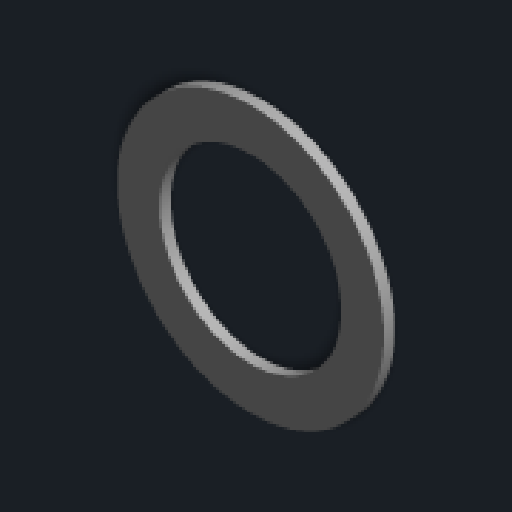
# Autodesk Inventor part: NeckRingAlign
Saved by Autodesk Inventor 2025.2 (Build 292293000, 293)
## iProperties
Created: 2025-09-16
Part Number: NeckRingAlign
Material: Generic
Document SubType Name: Sheet Metal
Designer: valer
Density: 1 g/cm^3
Sheet Metal Rule: Default_mm
Appearance: Default
Author: valer
Autodesk Inventor part; units mm, degrees
ref_plane "YZ Plane" through (0, 0, 0) normal (1, 0, 0) x (0, 1, 0)
ref_plane "XZ Plane" through (0, 0, 0) normal (0, 1, 0) x (-1, 0, 0)
ref_plane "XY Plane" through (0, 0, 0) normal (0, 0, 1) x (1, 0, 0)
sketch "Sketch1" plane through (0, 0, 0) normal (0, 0, 1) x (1, 0, 0)
  circle A0 centre (0, 0) radius 8.25
  circle A1 centre (0, 0) radius 15.621
  dimension "d1" = 16.5
  dimension "d2" = 31.242
  measures "d1" diameter of A0
  measures "d2" diameter of A1
extrude "Plate1" add sketch "Sketch1" along normal blind 3.175
sketch "Sketch2" plane through (0, 0, 0) normal (0, 0, -1) x (-1, 0, 0)
  circle A0 centre (-7.9638, -8.9766) radius 2 construction
  circle A1 centre (8.9766, -7.9638) radius 2 construction
  circle A2 centre (7.9638, 8.9766) radius 2 construction
  circle A3 centre (-8.9766, 7.9638) radius 2 construction
  circle A4 centre (-8.9766, 7.9638) radius 1.625
  circle A5 centre (7.9638, 8.9766) radius 1.625
  circle A6 centre (8.9766, -7.9638) radius 1.625
  circle A7 centre (-7.9638, -8.9766) radius 1.625
  point P0 (0, 0)
  dimension "d3" = 3.25
  constraints: 4 centre point, 4 coincident, 3 equal radius
  measures "d3" diameter of A4
extrude "Cut1" cut sketch "Sketch2" against normal blind 3.175
equation "\"d4\" = Thickness"
equation "\"d0\" = Thickness"
equation "\"BendRadius\" = Thickness"
equation "\"BendReliefWidth\" = Thickness"
equation "\"BendReliefDepth\" = 0.5 * Thickness"
equation "\"CornerReliefSize\" = 4 * Thickness"
equation "\"MinimumRemnant\" = 2 * Thickness"
equation "\"TransitionRadius\" = BendRadius"
equation "\"JacobiRadiusSize\" = BendRadius"
equation "\"GapSize\" = Thickness"
equation "\"Thickness\" = 3.175"
body "Solid1"
